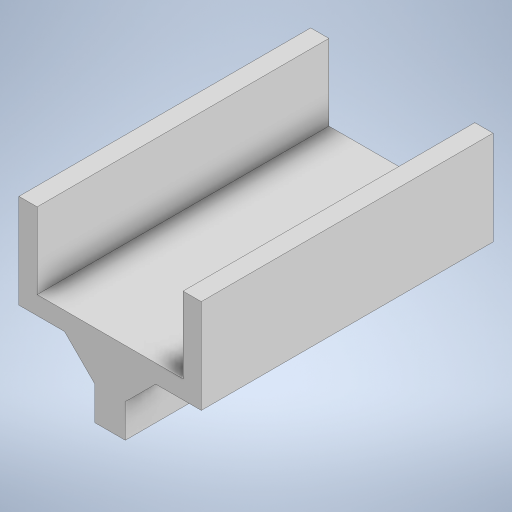
# Autodesk Inventor part: endcap_4mm_2ea_addon_large
Saved by Autodesk Inventor 2024 (Build 280153000, 153)
## iProperties
Created: 2024-04-25
Part Number: endcap_4mm_2ea_addon_large
Material: 일반
Document SubType Name: Modeling
Designer: Gihyeok Na
Density: 1 g/cm^3
Appearance: 기본값
Author: Gihyeok Na
Autodesk Inventor part; units mm, degrees
ref_plane "YZ Plane" through (0, 0, 0) normal (1, 0, 0) x (0, 1, 0)
ref_plane "XZ Plane" through (0, 0, 0) normal (0, 1, 0) x (-1, 0, 0)
ref_plane "XY Plane" through (0, 0, 0) normal (0, 0, 1) x (1, 0, 0)
sketch "스케치1" plane through (0, 0, 0) normal (0, 1, 0) x (-1, 0, 0)
  line L0 (-2.4, 4.8) -> (2.4, 4.8)
  line L1 (2.4, 4.8) -> (2.4, -4.8)
  line L2 (2.4, -4.8) -> (-2.4, -4.8)
  line L3 (-2.4, -4.8) -> (-2.4, 4.8)
  line L4 (-2.4, 4.8) -> (2.4, -4.8) construction
  line L5 (2.4, 4.8) -> (-2.4, -4.8) construction
  point P0 (0, 0)
  dimension "d0" = 4.8
  dimension "d1" = 9.6
  constraints: 12 end point, 2 midpoint, 2 parallel, 1 horizontal, 1 perpendicular
  measures "d0" distance of L1.end L2.end
  measures "d1" distance of L0.end L1.end
extrude "돌출1" add sketch "스케치1" along normal blind 0.6
sketch "스케치2" plane through (0, 0, 0) normal (0, -1, 0) x (1, 0, 0)
  line L0 (2.4, -4.8) -> (-2.4, -4.8) projected
  line L1 (2.4, 4.8) -> (2.4, -4.8) projected
  line L2 (-2.4, 4.8) -> (2.4, 4.8) projected
  line L3 (-2.4, -4.8) -> (-2.4, 4.8) projected
  line L4 (2.4, 4.8) -> (3, 4.8)
  line L5 (3, 4.8) -> (3, -4.8)
  line L6 (3, -4.8) -> (2.4, -4.8)
  line L7 (2.4, -4.8) -> (2.4, 4.8)
  line L8 (-2.4, -4.8) -> (-2.4, 4.8) projected
  line L9 (-2.4, 4.8) -> (-3, 4.8)
  line L10 (-3, 4.8) -> (-3, -4.8)
  line L11 (-3, -4.8) -> (-2.4, -4.8)
  line L12 (-2.4, -4.8) -> (-2.4, 4.8)
  point P0 (0, 0)
  dimension "d4" = 0.6
  dimension "d5" = 0.6
  constraints: 16 end point, 4 parallel, 2 horizontal, 2 perpendicular, 1 point on line
  measures "d4" distance of L5.end L6.end
  measures "d5" distance of L11.end L10.end
extrude "돌출2" add sketch "스케치2" against normal blind 3.1 contours L1 L4 L5 L6 | L11 L10 L9 L3
sketch "스케치3" plane through (0, 0, 0) normal (0, -1, 0) x (1, 0, 0)
  line L0 (2.4, -4.8) -> (-2.4, -4.8) projected
  line L1 (-0.5, 4.8) -> (0.5, 4.8)
  line L2 (0.5, 4.8) -> (0.5, -4.8)
  line L3 (0.5, -4.8) -> (-0.5, -4.8)
  line L4 (-0.5, -4.8) -> (-0.5, 4.8)
  line L5 (-0.5, 4.8) -> (0.5, -4.8) construction
  line L6 (0.5, 4.8) -> (-0.5, -4.8) construction
  point P0 (0, 0)
  dimension "d8" = 1
  constraints: 12 end point, 2 midpoint, 2 parallel, 1 horizontal, 1 perpendicular, 1 point on line
  measures "d8" distance of L2.end L3.end
extrude "돌출3" add sketch "스케치3" along normal blind 2.1
chamfer "모따기1" distance 1 angle 45 2 edges at (-0.5, 0, 0) (0.5, 0, 0)
sketch "스케치4" plane through (0, -2.1, 0) normal (0, -1, 0) x (1, 0, 0)
  line L0 (1.5, 4.8) -> (0.5, 4.8) projected
  line L1 (0.5, 4.8) -> (0.5, -4.8) projected
  line L2 (0.5, -4.8) -> (1.5, -4.8) projected
  line L3 (1.5, -4.8) -> (1.5, 4.8) projected
  line L4 (-0.5, 4.8) -> (-0.5, -4.8) projected
  line L5 (-0.5, -4.8) -> (0.5, -4.8) projected
  line L6 (0.5, -4.8) -> (0.5, 4.8) projected
  line L7 (0.5, 4.8) -> (-0.5, 4.8) projected
  line L8 (-1.5, -4.8) -> (-0.5, -4.8) projected
  line L9 (-0.5, -4.8) -> (-0.5, 4.8) projected
  line L10 (-0.5, 4.8) -> (-1.5, 4.8) projected
  line L11 (-1.5, 4.8) -> (-1.5, -4.8) projected
  line L12 (-1.5, 1.6) -> (1.5, 1.6)
  line L13 (1.5, 1.6) -> (1.5, -1.6)
  line L14 (1.5, -1.6) -> (-1.5, -1.6)
  line L15 (-1.5, -1.6) -> (-1.5, 1.6)
  line L16 (-1.5, 1.6) -> (1.5, -1.6) construction
  line L17 (1.5, 1.6) -> (-1.5, -1.6) construction
  point P0 (0, 0)
  point P1 (-0.5, -1.6)
  point P2 (-0.5, 1.6)
  point P3 (0.5, -1.6)
  point P4 (0.5, 1.6)
  dimension "d14" = 3.2
  constraints: 12 end point, 2 midpoint, 2 parallel, 1 horizontal, 1 perpendicular, 1 point on line
  measures "d14" distance of L12.end L13.end
extrude "돌출4" cut sketch "스케치4" against normal up to surface (2.1 mm away) contours L3 L14 L1 L12 | L4 L14 L11 L12
